# Autodesk Inventor part: clip_rod
Saved by Autodesk Inventor 2021 (Build 250183000, 183)
## iProperties
Created: 2021-03-20
Part Number: clip_rod
Material: ABS Plastic
Document SubType Name: Modeling
Designer: Tomasz Lisowski
Density: 1.06 g/cm^3
Appearance: Smooth - Black
Author: Tomasz Lisowski
Autodesk Inventor part; units mm, degrees
ref_plane "YZ Plane" through (0, 0, 0) normal (1, 0, 0) x (0, 1, 0)
ref_plane "XZ Plane" through (0, 0, 0) normal (0, 1, 0) x (-1, 0, 0)
ref_plane "XY Plane" through (0, 0, 0) normal (0, 0, 1) x (1, 0, 0)
sketch "Sketch1" plane through (0, 0, 0) normal (0, 1, 0) x (-1, 0, 0)
  circle A0 centre (0, 0) radius 4.1
  line L0 (6.3, 7.1) -> (-6.3, 7.1)
  line L1 (-6.3, 7.1) -> (-6.3, 5.1)
  line L2 (-6.3, 5.1) -> (6.3, 5.1)
  line L3 (6.3, 5.1) -> (6.3, 7.1)
  line L4 (6.3, 7.1) -> (-6.3, 5.1) construction
  line L5 (-6.3, 7.1) -> (6.3, 5.1) construction
  circle A1 centre (0, 0) radius 6.1
  line L6 (7.3, 8.1) -> (-7.3, 8.1)
  line L7 (-7.3, 8.1) -> (-7.3, 4.1)
  line L8 (-7.3, 4.1) -> (7.3, 4.1)
  line L9 (7.3, 4.1) -> (7.3, 8.1)
  point P0 (0, 6.1)
  point P1 (0, 6.1)
  point P2 (-4.5166, 4.1)
  point P3 (4.5166, 4.1)
  dimension "d0" = 8.2
  dimension "d1" = 12.6
  dimension "d2" = 2
  dimension "d3" = 1
  dimension "d4" = 1
  dimension "d5" = 2
  constraints: 20 end point, 4 parallel, 3 midpoint, 2 centre point, 2 coincident, 2 perpendicular, 1 horizontal, 1 vertical alignment, 3 other
  measures "d0" diameter of A0
  measures "d1" distance of L2.end L1.end
  measures "d2" distance of L1.end L0.end
  measures "d3" distance edge to line of A0 L2
  measures "d4" distance between parallel lines of L3 L9
  measures "d5" radial gap between concentric circles of A1 A0
extrude "Extrusion1" add sketch "Sketch1" along normal blind 4 contours L8 A1 | L8 A1 L2 | L8 L7 L6 L9 A1 L2 L3 L0 L1
fillet "Fillet1" radius 2 2 edges at (-4.5166, 2, 4.1) (4.5166, 2, 4.1)
fillet "Fillet2" radius 2 2 edges at (-7.3, 2, 4.1) (7.3, 2, 4.1)
fillet "Fillet3" radius 1 2 edges at (-7.3, 2, 8.1) (7.3, 2, 8.1)
sketch "Sketch2" plane through (0, 4, 0) normal (0, 1, 0) x (1, 0, 0)
  line L0 (6.3, -7.1) -> (-6.3, -7.1) projected
  line L1 (-6.3, -8.1) -> (6.3, -8.1) projected
  line L2 (-4.3, -7.1) -> (4.3, -7.1)
  line L3 (4.3, -7.1) -> (4.3, -8.1)
  line L4 (4.3, -8.1) -> (-4.3, -8.1)
  line L5 (-4.3, -8.1) -> (-4.3, -7.1)
  line L6 (-6.3, -7.1) -> (-6.3, -5.1) projected
  line L7 (6.3, -5.1) -> (6.3, -7.1) projected
  point P0 (0, 0)
  point P1 (4.3, -7.1)
  dimension "d11" = 2
  dimension "d12" = 2
  constraints: 8 end point, 2 parallel, 2 point on line, 1 horizontal, 1 perpendicular
  measures "d11" distance between parallel lines of L5 L6
  measures "d12" distance between parallel lines of L7 L3
extrude "Extrusion2" cut sketch "Sketch2" against normal through all
fillet "Fillet4" radius 0.5 4 edges at (-4.3, 2, 7.1) (-4.3, 2, 8.1) (4.3, 2, 7.1) (4.3, 2, 8.1)
fillet "Fillet5" radius 1 2 edges at (-6.3, 2, 7.1) (6.3, 2, 7.1)
fillet "Fillet6" radius 0.3 2 edges at (-6.3, 2, 5.1) (6.3, 2, 5.1)
body "Solid1"
